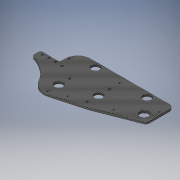
# Autodesk Inventor part: Flywheel Bracket 1
Saved by Autodesk Inventor 2019.4 (Build 234330000, 330)
## iProperties
Created: 2020-01-06
Part Number: Flywheel Bracket 1
Material: CFRP
Document SubType Name: Modeling
Designer: admin
Density: 1.43 g/cm^3
Appearance: Carbon Fiber
Mass: 153.476 g
Surface Area: 489.488 cm^2
Volume: 107.326 cm^3
Author: admin
Autodesk Inventor part; units mm, degrees
ref_plane "YZ Plane" through (0, 0, 0) normal (1, 0, 0) x (0, 1, 0)
ref_plane "XZ Plane" through (0, 0, 0) normal (0, 1, 0) x (-1, 0, 0)
ref_plane "XY Plane" through (0, 0, 0) normal (0, 0, 1) x (1, 0, 0)
sketch "Sketch1" plane through (0, 0, 0) normal (0, 1, 0) x (-1, 0, 0)
  circle A0 centre (-6.5438, 28.497) radius 9.5
  circle A1 centre (-6.5438, 28.497) radius 41.275 construction
  circle A2 centre (53.4562, 81.412) radius 9.5
  circle A3 centre (121.8221, 105.5441) radius 9.5
  circle A4 centre (113.4562, 28.497) radius 9.5
  circle A5 centre (113.4562, 28.497) radius 41.275 construction
  line L0 (113.4562, 28.497) -> (-6.5438, 28.497) construction
  circle A6 centre (53.4562, 81.412) radius 32.5 construction
  circle A7 centre (121.8221, 105.5441) radius 32.5 construction
  circle A8 centre (53.4562, -76.278) radius 88.9 construction
  line L1 (154.134, -76.278) -> (-96.866, -76.278) construction
  line L2 (121.8221, 105.5441) -> (53.4562, 81.412) construction
  line L3 (53.4562, 81.412) -> (-6.5438, 28.497) construction
  line L4 (121.8221, 105.5441) -> (113.4562, 28.497) construction
  line L5 (53.4562, 81.412) -> (113.4562, 28.497) construction
  line L6 (53.4562, 28.497) -> (53.4562, -76.278) construction
  line L7 (166.8221, 16.497) -> (-56.5438, 16.497)
  line L8 (-56.5438, 16.497) -> (-56.5438, 78.9049)
  line L9 (-56.5438, 78.9049) -> (41.6293, 117.0478)
  line L10 (41.6293, 117.0478) -> (141.6567, 144.7648)
  line L11 (141.6567, 144.7648) -> (166.8221, 78.722)
  line L12 (166.8221, 78.722) -> (210.9561, 78.722)
  line L13 (210.9561, 78.722) -> (210.9561, 58.722)
  line L14 (166.8221, 16.497) -> (166.8221, 58.722)
  line L15 (166.8221, 58.722) -> (210.9561, 58.722)
  line L16 (166.8221, 78.722) -> (166.8221, 58.722) construction
  circle A9 centre (53.4562, 81.412) radius 37.5 construction
  circle A10 centre (200.9561, 63.722) radius 2.75
  line L17 (200.9561, 63.722) -> (155.9561, 63.722) construction
  circle A11 centre (155.9561, 63.722) radius 2.75
  circle A12 centre (185.9561, 63.722) radius 2.75
  circle A13 centre (170.9561, 63.722) radius 2.75
  line L18 (53.4562, 56.012) -> (53.4562, 106.812) construction
  circle A14 centre (53.4562, 56.012) radius 2.75
  circle A15 centre (53.4562, 106.812) radius 2.75
  circle A16 centre (-51.5438, 44.497) radius 2.2
  circle A17 centre (6.3579, 92.6157) radius 2.2
  circle A18 centre (53.4562, 31.497) radius 2.2
  circle A19 centre (87.1568, 119.2864) radius 2.2
  circle A20 centre (160.8221, 41.497) radius 2.2
  line L19 (121.8221, 80.1441) -> (121.8221, 130.9441) construction
  circle A21 centre (121.8221, 80.1441) radius 2.75
  circle A22 centre (121.8221, 130.9441) radius 2.75
  circle A23 centre (-37.0438, 65.5611) radius 10.25
  circle A24 centre (-37.0438, 65.5611) radius 19.5 construction
  line L20 (-37.0438, 65.5611) -> (-6.5438, 28.497) construction
  circle A25 centre (-51.5438, 44.497) radius 5 construction
  circle A26 centre (-37.0438, 65.5611) radius 15 construction
  circle A27 centre (-37.0438, 80.5611) radius 1.65
  circle A28 centre (-50.0341, 58.0611) radius 1.65
  circle A29 centre (-24.0534, 58.0611) radius 1.65
  line L21 (-37.0438, 80.5611) -> (-37.0438, 65.5611) construction
  line L22 (-37.0438, 65.5611) -> (-50.0341, 58.0611) construction
  line L23 (-37.0438, 65.5611) -> (-24.0534, 58.0611) construction
  dimension "d67" = 19
  dimension "d68" = 82.55
  dimension "d69" = 19
  dimension "d70" = 19
  dimension "d71" = 19
  dimension "d72" = 82.55
  dimension "d73" = 65
  dimension "d74" = 65
  dimension "d75" = 120
  dimension "d76" = 177.8
  dimension "d77" = 104.775
  dimension "d78" = 80
  dimension "d79" = 80
  dimension "d80" = 77.5
  dimension "d81" = 72.5
  dimension "d82" = 12
  dimension "d83" = 50
  dimension "d85" = 75
  dimension "d86" = 20
  dimension "d87" = 44.134
  dimension "d88" = 5.5
  dimension "d90" = 5.5
  dimension "d91" = 5.5
  dimension "d93" = 15
  dimension "d95" = 5.5
  dimension "d96" = 15
  dimension "d97" = 15
  dimension "d98" = 5
  dimension "d99" = 10
  dimension "d100" = 135
  dimension "d105" = 45
  dimension "d106" = 50.8
  dimension "d107" = 5.5
  dimension "d108" = 5.5
  dimension "d112" = 4.4
  dimension "d114" = 4.4
  dimension "d115" = 4.4
  dimension "d116" = 4.4
  dimension "d117" = 4.4
  dimension "d118" = 6
  dimension "d119" = 25
  dimension "d120" = 15
  dimension "d121" = 110
  dimension "d122" = 10
  dimension "d123" = 10
  dimension "d124" = 60
  dimension "d125" = 145
  dimension "d127" = 5.5
  dimension "d128" = 5.5
  dimension "d129" = 50.8
  dimension "d132" = 20.5
  dimension "d133" = 39
  dimension "d134" = 48
  dimension "d135" = 10
  dimension "d136" = 28
  dimension "d137" = 30
  dimension "d138" = 3.3
  dimension "d139" = 3.3
  dimension "d140" = 3.3
  dimension "d141" = 120
  dimension "d142" = 120
  constraints: 49 end point, 30 centre point, 12 coincident, 7 tangent, 5 horizontal, 4 perpendicular, 4 vertical, 3 midpoint, 3 point on circle, 3 point on line, 1 parallel
  measures "d67" diameter of A0
  measures "d68" diameter of A1
  measures "d69" diameter of A2
  measures "d70" diameter of A3
  measures "d71" diameter of A4
  measures "d72" diameter of A5
  measures "d73" diameter of A6
  measures "d74" diameter of A7
  measures "d75" distance of L0.start L0.end
  measures "d76" diameter of A8
  measures "d77" distance between parallel lines of L1 L0
  measures "d78" distance of L2.end L0.end
  measures "d79" distance of L2.end L0.start
  measures "d80" distance of L2.start L0.start
  measures "d81" distance of L2.start L2.end
  measures "d82" distance from line of L7 A4.centre
  measures "d83" distance from line of A0.centre L8
  measures "d85" diameter of A9
  measures "d86" distance of L12.end L13.end
  measures "d87" distance of L11.end L12.end
  measures "d88" diameter of A10
  measures "d90" diameter of A11
  measures "d91" diameter of A12
  measures "d93" distance of A12.centre L17.start
  measures "d95" diameter of A13
  measures "d96" distance of A12.centre A13.centre
  measures "d97" distance of L17.end A13.centre
  measures "d98" distance from line of L15 L17.start
  measures "d99" distance from line of L13 L17.start
  measures "d100" distance between parallel lines of L1 L15
  measures "d105" distance from line of A3.centre L14
  measures "d106" distance of L18.start L18.end
  measures "d107" diameter of A14
  measures "d108" diameter of A15
  measures "d112" diameter of A16
  measures "d114" diameter of A17
  measures "d115" diameter of A18
  measures "d116" diameter of A19
  measures "d117" diameter of A20
  measures "d118" distance from line of L14 A20.centre
  measures "d119" distance from line of L7 A20.centre
  measures "d120" distance from line of L7 A18.centre
  measures "d121" distance from line of L8 A18.centre
  measures "d122" distance from line of L9 A17.centre
  measures "d123" distance from line of L10 A19.centre
  measures "d124" distance from line of L11 A19.centre
  measures "d125" distance from line of L11 A17.centre
  measures "d127" diameter of A21
  measures "d128" diameter of A22
  measures "d129" distance of L19.start L19.end
  measures "d132" diameter of A23
  measures "d133" diameter of A24
  measures "d134" distance of L20.start L0.end
  measures "d135" diameter of A25
  measures "d136" distance from line of L7 A16.centre
  measures "d137" diameter of A26
  measures "d138" diameter of A27
  measures "d139" diameter of A28
  measures "d140" diameter of A29
  measures "d141" angle of L21 L22
  measures "d142" angle of L21 L23
extrude "Extrusion1" add sketch "Sketch1" along normal blind 5
fillet "Fillet5" radius 10 2 edges at (56.5438, 2.5, 78.9049) (56.5438, 2.5, 16.497)
fillet "Fillet6" radius 37.5 1 edges at (-41.6293, 2.5, 117.0478)
fillet "Fillet7" radius 5 2 edges at (-210.9561, 2.5, 78.722) (-210.9561, 2.5, 58.722)
fillet "Fillet8" radius 100 1 edges at (-166.8221, 2.5, 78.722)
fillet "Fillet9" radius 32.5 1 edges at (-141.6567, 2.5, 144.7648)
fillet "Fillet10" radius 30 1 edges at (-166.8221, 2.5, 16.497)
fillet "Fillet11" radius 5 1 edges at (-166.8221, 2.5, 58.722)
body "Solid1"
